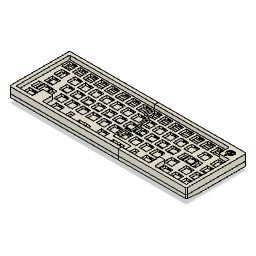
3d_print_case (Autodesk Fusion 360 design; units mm, degrees)
Autodesk Fusion 360 part; units mm, degrees
note: some values were not read from the file. Chosen so that the rebuilt part matches the saved one: which bodies a step acts on; which face or edge a step refers to. Set by a fixed rule: which sketch regions a step uses.
(part 1 of 3)
sketch "plate case top view" plane through (0, 0, 0) normal (0, 1, 0) x (1, 0, 0)
  line L0 (136.8258, 5.1029) -> (150.8248, 5.1029)
  line L1 (146.0628, 43.203) -> (132.0628, 43.203)
  line L2 (122.5378, 24.1528) -> (122.5378, 38.1522)
  line L3 (289.2258, 57.2023) -> (303.2248, 57.2023)
  line L4 (198.4498, 62.253) -> (184.4508, 62.253)
  line L5 (207.9748, 95.3023) -> (207.9748, 81.303)
  line L6 (284.1748, 95.3023) -> (284.1748, 81.303)
  line L7 (212.7378, 38.1522) -> (212.7378, 24.1528)
  line L8 (289.2258, 19.1023) -> (303.2248, 19.1023)
  line L9 (303.2248, 38.1522) -> (303.2248, 24.1528)
  line L10 (103.1998, 62.253) -> (89.2005, 62.253)
  line L11 (222.5508, 62.253) -> (222.5508, 76.2523)
  line L12 (231.7878, 19.1023) -> (231.7878, 5.1029)
  line L13 (265.1248, 95.3023) -> (265.1248, 81.303)
  line L14 (213.0258, 81.303) -> (213.0258, 95.3023)
  line L15 (303.2248, 62.253) -> (289.2258, 62.253)
  line L16 (193.9758, 81.303) -> (193.9758, 95.3023)
  line L17 (270.1758, 5.1029) -> (270.1758, 19.1023)
  line L18 (184.4508, 76.2523) -> (198.4498, 76.2523)
  line L19 (289.2258, 62.253) -> (289.2258, 76.2523)
  line L20 (246.0748, 95.3023) -> (246.0748, 81.303)
  line L21 (303.2248, 43.203) -> (289.2258, 43.203)
  line L22 (270.1758, 24.1528) -> (270.1758, 38.1522)
  line L23 (236.5498, 76.2523) -> (236.5498, 62.253)
  line L24 (79.6755, 95.3023) -> (93.6748, 95.3023)
  line L25 (179.3998, 76.2523) -> (179.3998, 62.253)
  line L26 (289.2258, 57.2023) -> (303.2248, 57.2023)
  line L27 (303.2248, 76.2523) -> (303.2248, 62.253)
  line L28 (203.2128, 43.203) -> (189.2128, 43.203)
  line L29 (188.9248, 95.3023) -> (188.9248, 81.303)
  line L30 (231.7878, 24.1528) -> (217.7878, 24.1528)
  line L31 (231.7878, 38.1522) -> (231.7878, 24.1528)
  line L32 (270.1758, 5.1029) -> (270.1758, 19.1023)
  line L33 (198.4498, 62.253) -> (184.4508, 62.253)
  line L34 (303.2248, 24.1528) -> (289.2258, 24.1528)
  line L35 (155.8758, 81.303) -> (155.8758, 95.3023)
  line L36 (217.7878, 38.1522) -> (231.7878, 38.1522)
  line L37 (203.5008, 76.2523) -> (217.4998, 76.2523)
  line L38 (232.0758, 81.303) -> (232.0758, 95.3023)
  line L39 (155.8758, 95.3023) -> (169.8748, 95.3023)
  line L40 (207.9748, 95.3023) -> (207.9748, 81.303)
  line L41 (284.1748, 5.1029) -> (270.1758, 5.1029)
  line L42 (284.1748, 19.1023) -> (284.1748, 5.1029)
  line L43 (189.2128, 57.2023) -> (203.2128, 57.2023)
  line L44 (303.2248, 62.253) -> (289.2258, 62.253)
  line L45 (303.2248, 5.1029) -> (289.2258, 5.1029)
  line L46 (241.6008, 76.2523) -> (255.5998, 76.2523)
  line L47 (222.5508, 62.253) -> (222.5508, 76.2523)
  line L48 (255.5998, 76.2523) -> (255.5998, 62.253)
  line L49 (289.2258, 62.253) -> (289.2258, 76.2523)
  line L50 (289.2258, 19.1023) -> (303.2248, 19.1023)
  line L51 (251.1258, 81.303) -> (251.1258, 95.3023)
  line L52 (270.1758, 81.303) -> (270.1758, 95.3023)
  line L53 (284.1748, 81.303) -> (270.1758, 81.303)
  line L54 (270.1758, 38.1522) -> (284.1748, 38.1522)
  line L55 (165.4008, 62.253) -> (165.4008, 76.2523)
  line L56 (303.2248, 5.1029) -> (289.2258, 5.1029)
  line L57 (251.1258, 81.303) -> (251.1258, 95.3023)
  line L58 (289.2258, 38.1522) -> (303.2248, 38.1522)
  line L59 (284.1748, 5.1029) -> (270.1758, 5.1029)
  line L60 (98.7241, 81.303) -> (98.7241, 95.3023)
  line L61 (270.1758, 19.1023) -> (284.1748, 19.1023)
  line L62 (89.2005, 76.2523) -> (103.1998, 76.2523)
  line L63 (79.6755, 81.303) -> (79.6755, 95.3023)
  line L64 (93.6748, 95.3023) -> (93.6748, 81.303)
  line L65 (93.6748, 81.303) -> (79.6755, 81.303)
  line L66 (255.5998, 62.253) -> (241.6008, 62.253)
  line L67 (270.1758, 95.3023) -> (284.1748, 95.3023)
  line L68 (188.9248, 81.303) -> (174.9258, 81.303)
  line L69 (289.2258, 24.1528) -> (289.2258, 38.1522)
  line L70 (265.4128, 62.253) -> (265.4128, 76.2523)
  line L71 (169.8748, 95.3023) -> (169.8748, 81.303)
  line L72 (74.913, 57.2023) -> (88.9123, 57.2023)
  line L73 (255.5998, 76.2523) -> (255.5998, 62.253)
  line L74 (207.9748, 81.303) -> (193.9758, 81.303)
  line L75 (270.1758, 19.1023) -> (284.1748, 19.1023)
  line L76 (289.2258, 5.1029) -> (289.2258, 19.1023)
  line L77 (279.4128, 62.253) -> (265.4128, 62.253)
  line L78 (222.2628, 43.203) -> (208.2628, 43.203)
  line L79 (265.4128, 62.253) -> (265.4128, 76.2523)
  line L80 (231.7878, 24.1528) -> (217.7878, 24.1528)
  line L81 (174.9258, 95.3023) -> (188.9248, 95.3023)
  line L82 (217.7878, 19.1023) -> (231.7878, 19.1023)
  line L83 (217.4998, 62.253) -> (203.5008, 62.253)
  line L84 (231.7878, 5.1029) -> (217.7878, 5.1029)
  line L85 (203.5008, 62.253) -> (203.5008, 76.2523)
  line L86 (155.8758, 95.3023) -> (169.8748, 95.3023)
  line L87 (217.4998, 62.253) -> (203.5008, 62.253)
  line L88 (231.7878, 5.1029) -> (217.7878, 5.1029)
  line L89 (303.2248, 76.2523) -> (303.2248, 62.253)
  line L90 (227.0248, 95.3023) -> (227.0248, 81.303)
  line L91 (284.1748, 19.1023) -> (284.1748, 5.1029)
  line L92 (279.4128, 76.2523) -> (279.4128, 62.253)
  line L93 (284.1748, 38.1522) -> (284.1748, 24.1528)
  line L94 (179.3998, 62.253) -> (165.4008, 62.253)
  line L95 (284.1748, 24.1528) -> (270.1758, 24.1528)
  line L96 (184.4508, 76.2523) -> (198.4498, 76.2523)
  line L97 (213.0258, 81.303) -> (213.0258, 95.3023)
  line L98 (198.4498, 76.2523) -> (198.4498, 62.253)
  line L99 (174.9258, 95.3023) -> (188.9248, 95.3023)
  line L100 (231.7878, 19.1023) -> (231.7878, 5.1029)
  line L101 (227.0248, 95.3023) -> (227.0248, 81.303)
  line L102 (289.2258, 76.2523) -> (303.2248, 76.2523)
  line L103 (208.2628, 57.2023) -> (222.2628, 57.2023)
  line L104 (174.9258, 81.303) -> (174.9258, 95.3023)
  line L105 (217.4998, 76.2523) -> (217.4998, 62.253)
  line L106 (212.7378, 24.1528) -> (198.7378, 24.1528)
  line L107 (93.6748, 95.3023) -> (93.6748, 81.303)
  line L108 (184.1628, 43.203) -> (170.1628, 43.203)
  line L109 (74.6248, 95.3023) -> (74.6248, 81.303)
  line L110 (103.1998, 62.253) -> (89.2005, 62.253)
  line L111 (79.6755, 81.303) -> (79.6755, 95.3023)
  line L112 (89.2005, 76.2523) -> (103.1998, 76.2523)
  line L113 (189.2128, 57.2023) -> (203.2128, 57.2023)
  line L114 (303.2248, 19.1023) -> (303.2248, 5.1029)
  line L115 (303.2248, 43.203) -> (289.2258, 43.203)
  line L116 (231.7878, 38.1522) -> (231.7878, 24.1528)
  line L117 (284.1748, 95.3023) -> (284.1748, 81.303)
  line L118 (217.4998, 76.2523) -> (217.4998, 62.253)
  line L119 (217.7878, 24.1528) -> (217.7878, 38.1522)
  line L120 (203.5008, 76.2523) -> (217.4998, 76.2523)
  line L121 (198.4498, 76.2523) -> (198.4498, 62.253)
  line L122 (279.4128, 62.253) -> (265.4128, 62.253)
  line L123 (213.0258, 95.3023) -> (227.0248, 95.3023)
  line L124 (217.7878, 19.1023) -> (231.7878, 19.1023)
  line L125 (289.2258, 76.2523) -> (303.2248, 76.2523)
  line L126 (169.8748, 95.3023) -> (169.8748, 81.303)
  line L127 (227.0248, 81.303) -> (213.0258, 81.303)
  line L128 (265.4128, 76.2523) -> (279.4128, 76.2523)
  line L129 (203.5008, 62.253) -> (203.5008, 76.2523)
  line L130 (169.8748, 81.303) -> (155.8758, 81.303)
  line L131 (169.8748, 81.303) -> (155.8758, 81.303)
  line L132 (212.7378, 38.1522) -> (212.7378, 24.1528)
  line L133 (265.1248, 95.3023) -> (265.1248, 81.303)
  line L134 (174.9258, 81.303) -> (174.9258, 95.3023)
  line L135 (303.2248, 38.1522) -> (303.2248, 24.1528)
  line L136 (212.7378, 24.1528) -> (198.7378, 24.1528)
  line L137 (246.0748, 95.3023) -> (246.0748, 81.303)
  line L138 (179.3998, 76.2523) -> (179.3998, 62.253)
  line L139 (303.2248, 19.1023) -> (303.2248, 5.1029)
  line L140 (193.9758, 95.3023) -> (207.9748, 95.3023)
  line L141 (289.2258, 5.1029) -> (289.2258, 19.1023)
  line L142 (155.8758, 81.303) -> (155.8758, 95.3023)
  line L143 (217.7878, 24.1528) -> (217.7878, 38.1522)
  line L144 (213.0258, 95.3023) -> (227.0248, 95.3023)
  line L145 (188.9248, 81.303) -> (174.9258, 81.303)
  line L146 (188.9248, 95.3023) -> (188.9248, 81.303)
  line L147 (270.1758, 81.303) -> (270.1758, 95.3023)
  line L148 (89.2005, 62.253) -> (89.2005, 76.2523)
  line L149 (74.913, 57.2023) -> (88.9123, 57.2023)
  line L150 (284.1748, 38.1522) -> (284.1748, 24.1528)
  line L151 (241.6008, 76.2523) -> (255.5998, 76.2523)
  line L152 (303.2248, 24.1528) -> (289.2258, 24.1528)
  line L153 (265.4128, 76.2523) -> (279.4128, 76.2523)
  line L154 (284.1748, 81.303) -> (270.1758, 81.303)
  line L155 (222.2628, 43.203) -> (208.2628, 43.203)
  line L156 (217.7878, 5.1029) -> (217.7878, 19.1023)
  line L157 (227.0248, 81.303) -> (213.0258, 81.303)
  line L158 (208.2628, 57.2023) -> (222.2628, 57.2023)
  line L159 (193.9758, 81.303) -> (193.9758, 95.3023)
  line L160 (279.4128, 76.2523) -> (279.4128, 62.253)
  line L161 (217.7878, 38.1522) -> (231.7878, 38.1522)
  line L162 (232.0758, 81.303) -> (232.0758, 95.3023)
  line L163 (217.7878, 5.1029) -> (217.7878, 19.1023)
  line L164 (270.1758, 95.3023) -> (284.1748, 95.3023)
  line L165 (255.5998, 62.253) -> (241.6008, 62.253)
  line L166 (198.7378, 38.1522) -> (212.7378, 38.1522)
  line L167 (170.1628, 57.2023) -> (184.1628, 57.2023)
  line L168 (203.2128, 43.203) -> (189.2128, 43.203)
  line L169 (89.2005, 62.253) -> (89.2005, 76.2523)
  line L170 (131.7748, 81.303) -> (117.7738, 81.303)
  line L171 (127.3008, 76.2523) -> (141.2998, 76.2523)
  line L172 (132.0628, 57.2023) -> (146.0628, 57.2023)
  line L173 (50.8123, 57.2023) -> (50.8123, 43.203)
  line L174 (108.2508, 62.253) -> (108.2508, 76.2523)
  line L175 (10.6178, 43.203) -> (10.6178, 57.2023)
  line L176 (69.8623, 5.1029) -> (55.863, 5.1029)
  line L177 (170.1628, 43.203) -> (170.1628, 57.2023)
  line L178 (107.9628, 57.2023) -> (107.9628, 43.203)
  line L179 (22.5255, 95.3023) -> (36.5248, 95.3023)
  line L180 (107.9628, 43.203) -> (93.963, 43.203)
  line L181 (46.338, 24.1528) -> (46.338, 38.1522)
  line L182 (88.9123, 57.2023) -> (88.9123, 43.203)
  line L183 (184.1628, 57.2023) -> (184.1628, 43.203)
  line L184 (51.1005, 62.253) -> (51.1005, 76.2523)
  line L185 (112.7248, 81.303) -> (98.7241, 81.303)
  line L186 (112.7248, 81.303) -> (98.7241, 81.303)
  line L187 (193.6878, 38.1522) -> (193.6878, 24.1528)
  line L188 (3.4754, 95.3023) -> (17.475, 95.3023)
  line L189 (289.2258, 24.1528) -> (289.2258, 38.1522)
  line L190 (241.6008, 62.253) -> (241.6008, 76.2523)
  line L191 (160.6378, 38.1522) -> (174.6378, 38.1522)
  line L192 (22.2375, 76.2523) -> (22.2375, 62.253)
  line L193 (243.9818, 24.1528) -> (243.9818, 38.1522)
  line L194 (65.0998, 76.2523) -> (65.0998, 62.253)
  line L195 (50.8123, 57.2023) -> (50.8123, 43.203)
  line L196 (32.0505, 62.253) -> (32.0505, 76.2523)
  line L197 (22.2375, 76.2523) -> (22.2375, 62.253)
  line L198 (65.0998, 76.2523) -> (65.0998, 62.253)
  line L199 (251.1258, 19.1023) -> (265.1248, 19.1023)
  line L200 (55.863, 57.2023) -> (69.8623, 57.2023)
  line L201 (22.5255, 81.303) -> (22.5255, 95.3023)
  line L202 (122.2498, 76.2523) -> (122.2498, 62.253)
  line L203 (243.9818, 38.1522) -> (257.9808, 38.1522)
  line L204 (55.5748, 81.303) -> (41.5755, 81.303)
  line L205 (29.3812, 38.1522) -> (15.3817, 38.1522)
  line L206 (60.3373, 24.1528) -> (46.338, 24.1528)
  line L207 (303.2248, 57.2023) -> (303.2248, 43.203)
  line L208 (165.1128, 57.2023) -> (165.1128, 43.203)
  line L209 (69.8623, 19.1023) -> (69.8623, 5.1029)
  line L210 (222.2628, 57.2023) -> (222.2628, 43.203)
  line L211 (55.863, 5.1029) -> (55.863, 19.1023)
  line L212 (46.338, 38.1522) -> (60.3373, 38.1522)
  line L213 (36.813, 57.2023) -> (50.8123, 57.2023)
  line L214 (170.1628, 43.203) -> (170.1628, 57.2023)
  line L215 (117.7738, 81.303) -> (117.7738, 95.3023)
  line L216 (303.2248, 57.2023) -> (303.2248, 43.203)
  line L217 (127.0128, 43.203) -> (113.0128, 43.203)
  line L218 (60.6255, 81.303) -> (60.6255, 95.3023)
  line L219 (265.1248, 19.1023) -> (265.1248, 5.1029)
  line L220 (132.0628, 57.2023) -> (146.0628, 57.2023)
  line L221 (32.0505, 76.2523) -> (46.0498, 76.2523)
  line L222 (222.2628, 57.2023) -> (222.2628, 43.203)
  line L223 (8.2379, 19.1023) -> (22.2375, 19.1023)
  line L224 (98.7241, 95.3023) -> (112.7248, 95.3023)
  line L225 (146.3508, 62.253) -> (146.3508, 76.2523)
  line L226 (222.5508, 76.2523) -> (236.5498, 76.2523)
  line L227 (65.388, 38.1522) -> (79.3873, 38.1522)
  line L228 (236.5498, 62.253) -> (222.5508, 62.253)
  line L229 (232.0758, 95.3023) -> (246.0748, 95.3023)
  line L230 (74.6248, 81.303) -> (60.6255, 81.303)
  line L231 (17.475, 95.3023) -> (17.475, 81.303)
  line L232 (265.1248, 5.1029) -> (251.1258, 5.1029)
  line L233 (184.1628, 57.2023) -> (184.1628, 43.203)
  line L234 (55.863, 5.1029) -> (55.863, 19.1023)
  line L235 (127.3008, 62.253) -> (127.3008, 76.2523)
  line L236 (113.0128, 57.2023) -> (127.0128, 57.2023)
  line L237 (36.813, 43.203) -> (36.813, 57.2023)
  line L238 (22.2375, 19.1023) -> (22.2375, 5.1029)
  line L239 (122.2498, 62.253) -> (108.2508, 62.253)
  line L240 (141.2998, 62.253) -> (127.3008, 62.253)
  line L241 (193.6878, 38.1522) -> (193.6878, 24.1528)
  line L242 (122.2498, 62.253) -> (108.2508, 62.253)
  line L243 (103.4878, 38.1522) -> (117.4878, 38.1522)
  line L244 (207.9748, 81.303) -> (193.9758, 81.303)
  line L245 (198.7378, 38.1522) -> (212.7378, 38.1522)
  line L246 (150.8248, 95.3023) -> (150.8248, 81.303)
  line L247 (146.3508, 76.2523) -> (160.3498, 76.2523)
  line L248 (127.0128, 43.203) -> (113.0128, 43.203)
  line L249 (236.5498, 62.253) -> (222.5508, 62.253)
  line L250 (79.3873, 24.1528) -> (65.388, 24.1528)
  line L251 (74.913, 43.203) -> (74.913, 57.2023)
  line L252 (246.0748, 81.303) -> (232.0758, 81.303)
  line L253 (74.913, 43.203) -> (74.913, 57.2023)
  line L254 (0.9508, 2.5769) -> (0.9508, 97.8267)
  line L255 (241.3128, 43.203) -> (227.3128, 43.203)
  line L256 (146.0628, 57.2023) -> (146.0628, 43.203)
  line L257 (151.1128, 43.203) -> (151.1128, 57.2023)
  line L258 (107.9628, 57.2023) -> (107.9628, 43.203)
  line L259 (246.0748, 81.303) -> (232.0758, 81.303)
  line L260 (227.3128, 57.2023) -> (241.3128, 57.2023)
  line L261 (232.0758, 95.3023) -> (246.0748, 95.3023)
  line L262 (127.0128, 57.2023) -> (127.0128, 43.203)
  line L263 (0.9508, 2.5769) -> (0.9508, 97.8267)
  line L264 (151.1128, 43.203) -> (151.1128, 57.2023)
  line L265 (227.3128, 43.203) -> (227.3128, 57.2023)
  line L266 (46.0498, 62.253) -> (32.0505, 62.253)
  line L267 (113.0128, 43.203) -> (113.0128, 57.2023)
  line L268 (93.963, 43.203) -> (93.963, 57.2023)
  line L269 (203.2128, 57.2023) -> (203.2128, 43.203)
  line L270 (36.5248, 81.303) -> (22.5255, 81.303)
  line L271 (257.9808, 38.1522) -> (257.9808, 24.1528)
  line L272 (165.4008, 76.2523) -> (179.3998, 76.2523)
  line L273 (65.388, 24.1528) -> (65.388, 38.1522)
  line L274 (103.4878, 38.1522) -> (117.4878, 38.1522)
  line L275 (79.6755, 95.3023) -> (93.6748, 95.3023)
  line L276 (165.4008, 76.2523) -> (179.3998, 76.2523)
  line L277 (93.963, 57.2023) -> (107.9628, 57.2023)
  line L278 (136.8258, 95.3023) -> (150.8248, 95.3023)
  line L279 (84.1498, 76.2523) -> (84.1498, 62.253)
  line L280 (127.3008, 76.2523) -> (141.2998, 76.2523)
  line L281 (160.3498, 76.2523) -> (160.3498, 62.253)
  line L282 (8.2379, 62.253) -> (8.2379, 76.2523)
  line L283 (22.2375, 62.253) -> (8.2379, 62.253)
  line L284 (155.5878, 38.1522) -> (155.5878, 24.1528)
  line L285 (55.863, 19.1023) -> (69.8623, 19.1023)
  line L286 (55.863, 57.2023) -> (69.8623, 57.2023)
  line L287 (8.2379, 76.2523) -> (22.2375, 76.2523)
  line L288 (24.6187, 57.2023) -> (24.6187, 43.203)
  line L289 (60.3373, 38.1522) -> (60.3373, 24.1528)
  line L290 (208.2628, 43.203) -> (208.2628, 57.2023)
  line L291 (127.3008, 62.253) -> (127.3008, 76.2523)
  line L292 (46.0498, 76.2523) -> (46.0498, 62.253)
  line L293 (136.5378, 24.1528) -> (122.5378, 24.1528)
  line L294 (265.1248, 81.303) -> (251.1258, 81.303)
  line L295 (22.5255, 81.303) -> (22.5255, 95.3023)
  line L296 (208.2628, 43.203) -> (208.2628, 57.2023)
  line L297 (55.5748, 81.303) -> (41.5755, 81.303)
  line L298 (60.6255, 95.3023) -> (74.6248, 95.3023)
  line L299 (241.3128, 43.203) -> (227.3128, 43.203)
  line L300 (41.5755, 95.3023) -> (55.5748, 95.3023)
  line L301 (193.6878, 24.1528) -> (179.6878, 24.1528)
  line L302 (24.6187, 43.203) -> (10.6178, 43.203)
  line L303 (65.0998, 62.253) -> (51.1005, 62.253)
  line L304 (222.5508, 76.2523) -> (236.5498, 76.2523)
  line L305 (65.388, 38.1522) -> (79.3873, 38.1522)
  line L306 (189.2128, 43.203) -> (189.2128, 57.2023)
  line L307 (69.8623, 19.1023) -> (69.8623, 5.1029)
  line L308 (193.9758, 95.3023) -> (207.9748, 95.3023)
  line L309 (136.8258, 81.303) -> (136.8258, 95.3023)
  line L310 (227.3128, 43.203) -> (227.3128, 57.2023)
  line L311 (117.7738, 95.3023) -> (131.7748, 95.3023)
  line L312 (108.2508, 76.2523) -> (122.2498, 76.2523)
  line L313 (65.0998, 62.253) -> (51.1005, 62.253)
  line L314 (198.7378, 24.1528) -> (198.7378, 38.1522)
  line L315 (243.9818, 38.1522) -> (257.9808, 38.1522)
  line L316 (69.8623, 57.2023) -> (69.8623, 43.203)
  line L317 (8.2379, 19.1023) -> (22.2375, 19.1023)
  line L318 (179.6878, 38.1522) -> (193.6878, 38.1522)
  line L319 (165.4008, 62.253) -> (165.4008, 76.2523)
  line L320 (103.1998, 76.2523) -> (103.1998, 62.253)
  line L321 (55.863, 43.203) -> (55.863, 57.2023)
  line L322 (22.2375, 5.1029) -> (8.2379, 5.1029)
  line L323 (122.5378, 24.1528) -> (122.5378, 38.1522)
  line L324 (160.3498, 62.253) -> (146.3508, 62.253)
  line L325 (146.3508, 76.2523) -> (160.3498, 76.2523)
  line L326 (0.9508, 97.8267) -> (305.7508, 97.8267)
  line L327 (305.7508, 2.5769) -> (0.9508, 2.5769)
  line L328 (165.1128, 43.203) -> (151.1128, 43.203)
  line L329 (305.7508, 2.5769) -> (0.9508, 2.5769)
  line L330 (155.5878, 24.1528) -> (141.5878, 24.1528)
  line L331 (70.1505, 76.2523) -> (84.1498, 76.2523)
  line L332 (151.1128, 57.2023) -> (165.1128, 57.2023)
  line L333 (141.5878, 38.1522) -> (155.5878, 38.1522)
  line L334 (50.8123, 43.203) -> (36.813, 43.203)
  line L335 (136.5378, 24.1528) -> (122.5378, 24.1528)
  line L336 (179.6878, 24.1528) -> (179.6878, 38.1522)
  line L337 (36.5248, 81.303) -> (22.5255, 81.303)
  line L338 (127.0128, 57.2023) -> (127.0128, 43.203)
  line L339 (131.7748, 95.3023) -> (131.7748, 81.303)
  line L340 (136.8258, 81.303) -> (136.8258, 95.3023)
  line L341 (60.6255, 81.303) -> (60.6255, 95.3023)
  line L342 (251.1258, 5.1029) -> (251.1258, 19.1023)
  line L343 (8.2379, 5.1029) -> (8.2379, 19.1023)
  line L344 (60.3373, 24.1528) -> (46.338, 24.1528)
  line L345 (46.338, 38.1522) -> (60.3373, 38.1522)
  line L346 (198.7378, 24.1528) -> (198.7378, 38.1522)
  line L347 (257.9808, 38.1522) -> (257.9808, 24.1528)
  line L348 (117.7738, 95.3023) -> (131.7748, 95.3023)
  line L349 (241.3128, 57.2023) -> (241.3128, 43.203)
  line L350 (132.0628, 43.203) -> (132.0628, 57.2023)
  line L351 (98.7241, 81.303) -> (98.7241, 95.3023)
  line L352 (179.3998, 62.253) -> (165.4008, 62.253)
  line L353 (15.3817, 24.1528) -> (29.3812, 24.1528)
  line L354 (251.1258, 95.3023) -> (265.1248, 95.3023)
  line L355 (70.1505, 62.253) -> (70.1505, 76.2523)
  line L356 (151.1128, 57.2023) -> (165.1128, 57.2023)
  line L357 (55.863, 19.1023) -> (69.8623, 19.1023)
  line L358 (41.5755, 81.303) -> (41.5755, 95.3023)
  line L359 (258.2678, 43.203) -> (272.2688, 43.203)
  line L360 (41.5755, 95.3023) -> (55.5748, 95.3023)
  line L361 (150.8248, 81.303) -> (136.8258, 81.303)
  line L362 (117.4878, 38.1522) -> (117.4878, 24.1528)
  line L363 (22.2375, 19.1023) -> (22.2375, 5.1029)
  line L364 (284.1748, 24.1528) -> (270.1758, 24.1528)
  line L365 (103.1998, 76.2523) -> (103.1998, 62.253)
  line L366 (93.963, 43.203) -> (93.963, 57.2023)
  line L367 (251.1258, 19.1023) -> (265.1248, 19.1023)
  line L368 (113.0128, 57.2023) -> (127.0128, 57.2023)
  line L369 (8.2379, 62.253) -> (8.2379, 76.2523)
  line L370 (69.8623, 57.2023) -> (69.8623, 43.203)
  line L371 (117.4878, 24.1528) -> (103.4878, 24.1528)
  line L372 (272.2688, 57.2023) -> (258.2678, 57.2023)
  line L373 (265.1248, 19.1023) -> (265.1248, 5.1029)
  line L374 (122.2498, 76.2523) -> (122.2498, 62.253)
  line L375 (193.6878, 24.1528) -> (179.6878, 24.1528)
  line L376 (257.9808, 24.1528) -> (243.9818, 24.1528)
  line L377 (17.475, 81.303) -> (3.4754, 81.303)
  line L378 (108.2508, 76.2523) -> (122.2498, 76.2523)
  line L379 (36.5248, 95.3023) -> (36.5248, 81.303)
  line L380 (146.3508, 62.253) -> (146.3508, 76.2523)
  line L381 (60.3373, 38.1522) -> (60.3373, 24.1528)
  line L382 (46.0498, 62.253) -> (32.0505, 62.253)
  line L383 (203.2128, 57.2023) -> (203.2128, 43.203)
  line L384 (179.6878, 38.1522) -> (193.6878, 38.1522)
  line L385 (174.6378, 24.1528) -> (160.6378, 24.1528)
  line L386 (107.9628, 43.203) -> (93.963, 43.203)
  line L387 (10.6178, 57.2023) -> (24.6187, 57.2023)
  line L388 (174.6378, 38.1522) -> (174.6378, 24.1528)
  line L389 (55.5748, 95.3023) -> (55.5748, 81.303)
  line L390 (36.813, 57.2023) -> (50.8123, 57.2023)
  line L391 (305.7508, 97.8267) -> (305.7508, 2.5769)
  line L392 (251.1258, 5.1029) -> (251.1258, 19.1023)
  line L393 (22.2375, 5.1029) -> (8.2379, 5.1029)
  line L394 (113.0128, 43.203) -> (113.0128, 57.2023)
  line L395 (88.9123, 57.2023) -> (88.9123, 43.203)
  line L396 (70.1505, 62.253) -> (70.1505, 76.2523)
  line L397 (305.7508, 97.8267) -> (305.7508, 2.5769)
  line L398 (32.0505, 76.2523) -> (46.0498, 76.2523)
  line L399 (98.7241, 95.3023) -> (112.7248, 95.3023)
  line L400 (174.6378, 24.1528) -> (160.6378, 24.1528)
  line L401 (15.3817, 24.1528) -> (29.3812, 24.1528)
  line L402 (69.8623, 43.203) -> (55.863, 43.203)
  line L403 (160.6378, 24.1528) -> (160.6378, 38.1522)
  line L404 (189.2128, 43.203) -> (189.2128, 57.2023)
  line L405 (174.6378, 38.1522) -> (174.6378, 24.1528)
  line L406 (79.3873, 24.1528) -> (65.388, 24.1528)
  line L407 (51.1005, 62.253) -> (51.1005, 76.2523)
  line L408 (55.863, 43.203) -> (55.863, 57.2023)
  line L409 (84.1498, 62.253) -> (70.1505, 62.253)
  line L410 (84.1498, 62.253) -> (70.1505, 62.253)
  line L411 (141.2998, 76.2523) -> (141.2998, 62.253)
  line L412 (17.475, 95.3023) -> (17.475, 81.303)
  line L413 (289.2258, 43.203) -> (289.2258, 57.2023)
  line L414 (258.2678, 43.203) -> (272.2688, 43.203)
  line L415 (60.6255, 95.3023) -> (74.6248, 95.3023)
  line L416 (70.1505, 76.2523) -> (84.1498, 76.2523)
  line L417 (46.338, 24.1528) -> (46.338, 38.1522)
  line L418 (146.0628, 57.2023) -> (146.0628, 43.203)
  line L419 (22.5255, 95.3023) -> (36.5248, 95.3023)
  line L420 (69.8623, 5.1029) -> (55.863, 5.1029)
  line L421 (3.4754, 81.303) -> (3.4754, 95.3023)
  line L422 (17.475, 81.303) -> (3.4754, 81.303)
  line L423 (8.2379, 76.2523) -> (22.2375, 76.2523)
  line L424 (289.2258, 43.203) -> (289.2258, 57.2023)
  line L425 (29.3812, 38.1522) -> (15.3817, 38.1522)
  line L426 (141.2998, 76.2523) -> (141.2998, 62.253)
  line L427 (131.7748, 81.303) -> (117.7738, 81.303)
  line L428 (46.0498, 76.2523) -> (46.0498, 62.253)
  line L429 (10.6178, 43.203) -> (10.6178, 57.2023)
  line L430 (160.6378, 38.1522) -> (174.6378, 38.1522)
  line L431 (65.388, 24.1528) -> (65.388, 38.1522)
  line L432 (8.2379, 5.1029) -> (8.2379, 19.1023)
  line L433 (272.2688, 57.2023) -> (258.2678, 57.2023)
  line L434 (112.7248, 95.3023) -> (112.7248, 81.303)
  line L435 (108.2508, 62.253) -> (108.2508, 76.2523)
  line L436 (112.7248, 95.3023) -> (112.7248, 81.303)
  line L437 (117.7738, 81.303) -> (117.7738, 95.3023)
  line L438 (289.2258, 38.1522) -> (303.2248, 38.1522)
  line L439 (55.5748, 95.3023) -> (55.5748, 81.303)
  line L440 (3.4754, 95.3023) -> (17.475, 95.3023)
  line L441 (24.6187, 43.203) -> (10.6178, 43.203)
  line L442 (69.8623, 43.203) -> (55.863, 43.203)
  line L443 (251.1258, 95.3023) -> (265.1248, 95.3023)
  line L444 (160.3498, 76.2523) -> (160.3498, 62.253)
  line L445 (170.1628, 57.2023) -> (184.1628, 57.2023)
  line L446 (141.2998, 62.253) -> (127.3008, 62.253)
  line L447 (74.6248, 81.303) -> (60.6255, 81.303)
  line L448 (227.3128, 57.2023) -> (241.3128, 57.2023)
  line L449 (122.5378, 38.1522) -> (136.5378, 38.1522)
  line L450 (3.4754, 81.303) -> (3.4754, 95.3023)
  line L451 (36.5248, 95.3023) -> (36.5248, 81.303)
  line L452 (36.813, 43.203) -> (36.813, 57.2023)
  line L453 (22.2375, 62.253) -> (8.2379, 62.253)
  line L454 (243.9818, 24.1528) -> (243.9818, 38.1522)
  line L455 (165.1128, 57.2023) -> (165.1128, 43.203)
  line L456 (51.1005, 76.2523) -> (65.0998, 76.2523)
  line L457 (150.8248, 95.3023) -> (150.8248, 81.303)
  line L458 (155.5878, 38.1522) -> (155.5878, 24.1528)
  line L459 (165.1128, 43.203) -> (151.1128, 43.203)
  line L460 (160.6378, 24.1528) -> (160.6378, 38.1522)
  line L461 (10.6178, 57.2023) -> (24.6187, 57.2023)
  line L462 (117.4878, 24.1528) -> (103.4878, 24.1528)
  line L463 (50.8123, 43.203) -> (36.813, 43.203)
  line L464 (184.4508, 62.253) -> (184.4508, 76.2523)
  line L465 (179.6878, 24.1528) -> (179.6878, 38.1522)
  line L466 (93.6748, 81.303) -> (79.6755, 81.303)
  line L467 (32.0505, 62.253) -> (32.0505, 76.2523)
  line L468 (117.4878, 38.1522) -> (117.4878, 24.1528)
  line L469 (131.7748, 95.3023) -> (131.7748, 81.303)
  line L470 (150.8248, 81.303) -> (136.8258, 81.303)
  line L471 (241.6008, 62.253) -> (241.6008, 76.2523)
  line L472 (74.6248, 95.3023) -> (74.6248, 81.303)
  line L473 (84.1498, 76.2523) -> (84.1498, 62.253)
  line L474 (132.0628, 43.203) -> (132.0628, 57.2023)
  line L475 (241.3128, 57.2023) -> (241.3128, 43.203)
  line L476 (257.9808, 24.1528) -> (243.9818, 24.1528)
  line L477 (24.6187, 57.2023) -> (24.6187, 43.203)
  line L478 (270.1758, 24.1528) -> (270.1758, 38.1522)
  line L479 (236.5498, 76.2523) -> (236.5498, 62.253)
  line L480 (184.1628, 43.203) -> (170.1628, 43.203)
  line L481 (41.5755, 81.303) -> (41.5755, 95.3023)
  line L482 (265.1248, 81.303) -> (251.1258, 81.303)
  line L483 (136.8258, 95.3023) -> (150.8248, 95.3023)
  line L484 (93.963, 57.2023) -> (107.9628, 57.2023)
  line L485 (51.1005, 76.2523) -> (65.0998, 76.2523)
  line L486 (270.1758, 38.1522) -> (284.1748, 38.1522)
  line L487 (184.4508, 62.253) -> (184.4508, 76.2523)
  line L488 (265.1248, 5.1029) -> (251.1258, 5.1029)
  line L489 (155.5878, 24.1528) -> (141.5878, 24.1528)
  line L490 (136.5378, 38.1522) -> (136.5378, 24.1528)
  line L491 (136.8258, 5.1029) -> (150.8248, 5.1029)
  line L492 (150.8248, 19.1023) -> (136.8258, 19.1023)
  line L493 (84.438, 38.1522) -> (98.4373, 38.1522)
  line L494 (146.0628, 43.203) -> (132.0628, 43.203)
  line L495 (98.4373, 38.1522) -> (98.4373, 24.1528)
  line L496 (88.9123, 43.203) -> (74.913, 43.203)
  line L497 (141.5878, 24.1528) -> (141.5878, 38.1522)
  line L498 (79.3873, 38.1522) -> (79.3873, 24.1528)
  line L499 (150.8248, 19.1023) -> (136.8258, 19.1023)
  line L500 (136.5378, 38.1522) -> (136.5378, 24.1528)
  line L501 (122.5378, 38.1522) -> (136.5378, 38.1522)
  line L502 (84.438, 24.1528) -> (84.438, 38.1522)
  line L503 (98.4373, 24.1528) -> (84.438, 24.1528)
  line L504 (98.4373, 38.1522) -> (98.4373, 24.1528)
  line L505 (84.438, 24.1528) -> (84.438, 38.1522)
  line L506 (141.5878, 24.1528) -> (141.5878, 38.1522)
  line L507 (84.438, 38.1522) -> (98.4373, 38.1522)
  line L508 (103.4878, 24.1528) -> (103.4878, 38.1522)
  line L509 (79.3873, 38.1522) -> (79.3873, 24.1528)
  line L510 (0.9508, 97.8267) -> (305.7508, 97.8267)
  line L511 (103.4878, 24.1528) -> (103.4878, 38.1522)
  line L512 (88.9123, 43.203) -> (74.913, 43.203)
  line L513 (160.3498, 62.253) -> (146.3508, 62.253)
  line L514 (141.5878, 38.1522) -> (155.5878, 38.1522)
  line L515 (98.4373, 24.1528) -> (84.438, 24.1528)
  line L516 (13.8562, 37.604) -> (13.8562, 23.4018)
  line L517 (6.2811, 23.4018) -> (6.2811, 37.604)
  line L518 (15.3817, 38.1522) -> (15.3817, 24.1528)
  line L519 (6.2811, 37.604) -> (13.8562, 37.604)
  line L520 (6.2811, 23.4018) -> (13.8562, 23.4018)
  line L521 (30.9067, 37.604) -> (38.4817, 37.604)
  line L522 (38.4817, 37.604) -> (38.4817, 23.4018)
  line L523 (30.9067, 23.4018) -> (30.9067, 37.604)
  line L524 (29.3812, 38.1522) -> (29.3812, 24.1528)
  line L525 (30.9067, 23.4018) -> (38.4817, 23.4018)
  line L526 (256.7438, 56.6526) -> (256.7438, 42.4519)
  line L527 (256.7438, 42.4519) -> (249.1688, 42.4519)
  line L528 (249.1688, 42.4519) -> (249.1688, 56.6526)
  line L529 (258.2678, 57.2023) -> (258.2678, 43.203)
  line L530 (249.1688, 56.6526) -> (256.7438, 56.6526)
  line L531 (281.3678, 56.6526) -> (273.7928, 56.6526)
  line L532 (273.7928, 56.6526) -> (273.7928, 42.4519)
  line L533 (273.7928, 42.4519) -> (281.3678, 42.4519)
  line L534 (281.3678, 42.4519) -> (281.3678, 56.6526)
  line L535 (272.2688, 57.2023) -> (272.2688, 43.203)
  line L536 (205.1748, 18.5539) -> (197.5998, 18.5539)
  line L537 (197.5998, 18.5539) -> (197.5998, 4.3518)
  line L538 (197.5998, 4.3518) -> (205.1748, 4.3518)
  line L539 (205.1748, 4.3518) -> (205.1748, 18.5539)
  line L540 (82.4755, 18.5539) -> (90.0507, 18.5539)
  line L541 (90.0507, 18.5539) -> (90.0507, 4.3518)
  line L542 (90.0507, 4.3518) -> (82.4755, 4.3518)
  line L543 (82.4755, 4.3518) -> (82.4755, 18.5539)
  line L544 (150.8248, 19.1023) -> (150.8248, 5.1029)
  line L545 (136.8258, 19.1023) -> (136.8258, 5.1029)
  circle A0 centre (113.4382, 11.4529) radius 3
  line L546 (123.4382, 11.4529) -> (123.4382, 13.4529)
  line L547 (123.4382, 13.4529) -> (113.4382, 13.4529)
  line L548 (123.4382, 11.4529) -> (123.4382, 9.4529)
  line L549 (123.4382, 9.4529) -> (113.4382, 9.4529)
  line L550 (103.4382, 11.4529) -> (103.4382, 13.4529)
  line L551 (103.4382, 13.4529) -> (113.4382, 13.4529)
  line L552 (103.4382, 11.4529) -> (103.4382, 9.4529)
  line L553 (103.4382, 9.4529) -> (113.4382, 9.4529)
  line L554 (184.2123, 13.4529) -> (174.2123, 13.4529)
  line L555 (164.2123, 13.4529) -> (174.2123, 13.4529)
  line L556 (164.2123, 11.4529) -> (164.2123, 9.4529)
  line L557 (164.2123, 11.4529) -> (164.2123, 13.4529)
  line L558 (164.2123, 9.4529) -> (174.2123, 9.4529)
  line L559 (184.2123, 11.4529) -> (184.2123, 9.4529)
  circle A1 centre (174.2123, 11.4529) radius 3
  line L560 (184.2123, 9.4529) -> (174.2123, 9.4529)
  line L561 (184.2123, 11.4529) -> (184.2123, 13.4529)
  line L562 (306.1758, 2.1519) -> (0.5258, 2.1519)
  line L563 (0.5258, 2.1519) -> (0.5258, 98.2517)
  line L564 (0.5258, 98.2517) -> (306.1758, 98.2517)
  line L565 (306.1758, 98.2517) -> (306.1758, 2.1519)
  line L566 (312.1758, -3.8481) -> (-5.4742, -3.8481)
  line L567 (-5.4742, -3.8481) -> (-5.4742, 104.2517)
  line L568 (-5.4742, 104.2517) -> (312.1758, 104.2517)
  line L569 (312.1758, 104.2517) -> (312.1758, -3.8481)
  line L570 (30.0505, 3.1029) -> (30.0505, 21.1023)
  line L571 (30.0505, 21.1023) -> (48.0498, 21.1023)
  line L572 (48.0498, 21.1023) -> (48.0498, 3.1029)
  line L573 (30.0505, 3.1029) -> (30.0505, 2.1519)
  line L574 (48.0498, 3.1029) -> (48.0498, 2.1519)
  line L575 (249.1258, 21.1023) -> (239.6008, 21.1023)
  line L576 (239.6008, 21.1023) -> (239.6008, 2.1519)
  line L577 (249.1258, 21.1023) -> (249.1258, 2.1519)
  line L578 (287.2258, 98.2517) -> (306.1758, 98.2517)
  line L579 (306.1758, 98.2517) -> (306.1758, 79.303)
  line L580 (306.1758, 79.303) -> (287.2258, 79.303)
  line L581 (287.2258, 79.303) -> (287.2258, 98.2517)
  constraint coincident L562 L573.end
  constraint coincident L562 L574.end
  constraint coincident L562 L576.end
  constraint coincident L562 L577.end
  constraint coincident L565 L579.end
  constraint coincident L564 L578.start
extrude "Extrude1" add sketch "plate case top view" against normal blind 4 contours L254 L263 L326 L327 L329 L510 L562 L563 L564 L573 L581 | L254 L263 L326 L327 L329 L391 L397 L510 L570 L571 L572 L573 L574 L575 L576 L577 L580 L581 | L327 L329 L570 L571 L572 L573 L574 | L327 L329 L562 L573 L574 | L326 L391 L397 L510 L564 L565 L578 L579 L580 L581 | L326 L391 L397 L510 L580 L581 | L327 L329 L562 L574 L576 | L327 L329 L575 L576 L577 | L327 L329 L562 L576 L577 | L327 L329 L391 L397 L562 L565 L577 L580 | L566 L567 L568 L569 makes body 1
extrude "Extrude2" add sketch "plate case top view" along normal blind 7 contours L327 L329 L570 L571 L572 L573 L574 | L327 L329 L562 L573 L574 | L326 L391 L397 L510 L564 L565 L578 L579 L580 L581 | L326 L391 L397 L510 L580 L581 | L327 L329 L575 L576 L577 | L327 L329 L562 L576 L577 | L566 L567 L568 L569 bodies 1
sketch "plate switch clips" plane through (0, -4, 0) normal (0, -1, 0) x (1, 0, 0)
  line L0 (98.4373, -24.1528) -> (98.4373, -38.1522)
  line L1 (98.4373, -38.1522) -> (84.438, -38.1522)
  line L2 (84.438, -38.1522) -> (84.438, -24.1528)
  line L3 (84.438, -24.1528) -> (98.4373, -24.1528)
  line L4 (3.4754, -81.303) -> (17.475, -81.303)
  line L5 (17.475, -81.303) -> (17.475, -95.3023)
  line L6 (17.475, -95.3023) -> (3.4754, -95.3023)
  line L7 (3.4754, -95.3023) -> (3.4754, -81.303)
  line L8 (279.4128, -76.2523) -> (265.4128, -76.2523)
  line L9 (265.4128, -76.2523) -> (265.4128, -62.253)
  line L10 (265.4128, -62.253) -> (279.4128, -62.253)
  line L11 (279.4128, -62.253) -> (279.4128, -76.2523)
  line L12 (51.1005, -76.2523) -> (51.1005, -62.253)
  line L13 (51.1005, -62.253) -> (65.0998, -62.253)
  line L14 (65.0998, -62.253) -> (65.0998, -76.2523)
  line L15 (65.0998, -76.2523) -> (51.1005, -76.2523)
  line L16 (270.1758, -38.1522) -> (270.1758, -24.1528)
  line L17 (270.1758, -24.1528) -> (284.1748, -24.1528)
  line L18 (284.1748, -24.1528) -> (284.1748, -38.1522)
  line L19 (284.1748, -38.1522) -> (270.1758, -38.1522)
  line L20 (103.4878, -24.1528) -> (117.4878, -24.1528)
  line L21 (117.4878, -24.1528) -> (117.4878, -38.1522)
  line L22 (117.4878, -38.1522) -> (103.4878, -38.1522)
  line L23 (103.4878, -38.1522) -> (103.4878, -24.1528)
  line L24 (141.5878, -38.1522) -> (141.5878, -24.1528)
  line L25 (141.5878, -24.1528) -> (155.5878, -24.1528)
  line L26 (155.5878, -24.1528) -> (155.5878, -38.1522)
  line L27 (155.5878, -38.1522) -> (141.5878, -38.1522)
  line L28 (179.6878, -24.1528) -> (193.6878, -24.1528)
  line L29 (193.6878, -24.1528) -> (193.6878, -38.1522)
  line L30 (193.6878, -38.1522) -> (179.6878, -38.1522)
  line L31 (179.6878, -38.1522) -> (179.6878, -24.1528)
  line L32 (141.2998, -62.253) -> (141.2998, -76.2523)
  line L33 (141.2998, -76.2523) -> (127.3008, -76.2523)
  line L34 (127.3008, -76.2523) -> (127.3008, -62.253)
  line L35 (127.3008, -62.253) -> (141.2998, -62.253)
  line L36 (281.3678, -42.4519) -> (281.3678, -56.6526)
  line L37 (281.3678, -56.6526) -> (273.7928, -56.6526)
  line L38 (273.7928, -56.6526) -> (273.7928, -42.4519)
  line L39 (273.7928, -42.4519) -> (281.3678, -42.4519)
  line L40 (112.7248, -95.3023) -> (98.7241, -95.3023)
  line L41 (98.7241, -95.3023) -> (98.7241, -81.303)
  line L42 (98.7241, -81.303) -> (112.7248, -81.303)
  line L43 (112.7248, -81.303) -> (112.7248, -95.3023)
  line L44 (258.2678, -57.2023) -> (258.2678, -43.203)
  line L45 (258.2678, -43.203) -> (272.2688, -43.203)
  line L46 (272.2688, -43.203) -> (272.2688, -57.2023)
  line L47 (272.2688, -57.2023) -> (258.2678, -57.2023)
  line L48 (8.2379, -5.1029) -> (22.2375, -5.1029)
  line L49 (22.2375, -5.1029) -> (22.2375, -19.1023)
  line L50 (22.2375, -19.1023) -> (8.2379, -19.1023)
  line L51 (8.2379, -19.1023) -> (8.2379, -5.1029)
  line L52 (108.2508, -62.253) -> (122.2498, -62.253)
  line L53 (122.2498, -62.253) -> (122.2498, -76.2523)
  line L54 (122.2498, -76.2523) -> (108.2508, -76.2523)
  line L55 (108.2508, -76.2523) -> (108.2508, -62.253)
  line L56 (188.9248, -95.3023) -> (174.9258, -95.3023)
  line L57 (174.9258, -95.3023) -> (174.9258, -81.303)
  line L58 (174.9258, -81.303) -> (188.9248, -81.303)
  line L59 (188.9248, -81.303) -> (188.9248, -95.3023)
  line L60 (22.2375, -62.253) -> (22.2375, -76.2523)
  line L61 (22.2375, -76.2523) -> (8.2379, -76.2523)
  line L62 (8.2379, -76.2523) -> (8.2379, -62.253)
  line L63 (8.2379, -62.253) -> (22.2375, -62.253)
  line L64 (284.1748, -19.1023) -> (270.1758, -19.1023)
  line L65 (270.1758, -19.1023) -> (270.1758, -5.1029)
  line L66 (270.1758, -5.1029) -> (284.1748, -5.1029)
  line L67 (284.1748, -5.1029) -> (284.1748, -19.1023)
  line L68 (165.1128, -43.203) -> (165.1128, -57.2023)
  line L69 (165.1128, -57.2023) -> (151.1128, -57.2023)
  line L70 (151.1128, -57.2023) -> (151.1128, -43.203)
  line L71 (151.1128, -43.203) -> (165.1128, -43.203)
  line L72 (193.9758, -95.3023) -> (193.9758, -81.303)
  line L73 (193.9758, -81.303) -> (207.9748, -81.303)
  line L74 (207.9748, -81.303) -> (207.9748, -95.3023)
  line L75 (207.9748, -95.3023) -> (193.9758, -95.3023)
  line L76 (289.2258, -5.1029) -> (303.2248, -5.1029)
  line L77 (303.2248, -5.1029) -> (303.2248, -19.1023)
  line L78 (303.2248, -19.1023) -> (289.2258, -19.1023)
  line L79 (289.2258, -19.1023) -> (289.2258, -5.1029)
  line L80 (289.2258, -76.2523) -> (289.2258, -62.253)
  line L81 (289.2258, -62.253) -> (303.2248, -62.253)
  line L82 (303.2248, -62.253) -> (303.2248, -76.2523)
  line L83 (303.2248, -76.2523) -> (289.2258, -76.2523)
  line L84 (69.8623, -43.203) -> (69.8623, -57.2023)
  line L85 (69.8623, -57.2023) -> (55.863, -57.2023)
  line L86 (55.863, -57.2023) -> (55.863, -43.203)
  line L87 (55.863, -43.203) -> (69.8623, -43.203)
  line L88 (189.2128, -43.203) -> (203.2128, -43.203)
  line L89 (203.2128, -43.203) -> (203.2128, -57.2023)
  line L90 (203.2128, -57.2023) -> (189.2128, -57.2023)
  line L91 (189.2128, -57.2023) -> (189.2128, -43.203)
  line L92 (249.1688, -56.6526) -> (249.1688, -42.4519)
  line L93 (249.1688, -42.4519) -> (256.7438, -42.4519)
  line L94 (256.7438, -42.4519) -> (256.7438, -56.6526)
  line L95 (256.7438, -56.6526) -> (249.1688, -56.6526)
  line L96 (46.338, -24.1528) -> (60.3373, -24.1528)
  line L97 (60.3373, -24.1528) -> (60.3373, -38.1522)
  line L98 (60.3373, -38.1522) -> (46.338, -38.1522)
  line L99 (46.338, -38.1522) -> (46.338, -24.1528)
  line L100 (270.1758, -95.3023) -> (270.1758, -81.303)
  line L101 (270.1758, -81.303) -> (284.1748, -81.303)
  line L102 (284.1748, -81.303) -> (284.1748, -95.3023)
  line L103 (284.1748, -95.3023) -> (270.1758, -95.3023)
  line L104 (15.3817, -38.1522) -> (15.3817, -24.1528)
  line L105 (15.3817, -24.1528) -> (29.3812, -24.1528)
  line L106 (29.3812, -24.1528) -> (29.3812, -38.1522)
  line L107 (29.3812, -38.1522) -> (15.3817, -38.1522)
  line L108 (79.3873, -38.1522) -> (65.388, -38.1522)
  line L109 (65.388, -38.1522) -> (65.388, -24.1528)
  line L110 (65.388, -24.1528) -> (79.3873, -24.1528)
  line L111 (79.3873, -24.1528) -> (79.3873, -38.1522)
  line L112 (30.9067, -37.604) -> (30.9067, -23.4018)
  line L113 (30.9067, -23.4018) -> (38.4817, -23.4018)
  line L114 (38.4817, -23.4018) -> (38.4817, -37.604)
  line L115 (38.4817, -37.604) -> (30.9067, -37.604)
  line L116 (50.8123, -43.203) -> (50.8123, -57.2023)
  line L117 (50.8123, -57.2023) -> (36.813, -57.2023)
  line L118 (36.813, -57.2023) -> (36.813, -43.203)
  line L119 (36.813, -43.203) -> (50.8123, -43.203)
  line L120 (88.9123, -43.203) -> (88.9123, -57.2023)
  line L121 (88.9123, -57.2023) -> (74.913, -57.2023)
  line L122 (74.913, -57.2023) -> (74.913, -43.203)
  line L123 (74.913, -43.203) -> (88.9123, -43.203)
  line L124 (32.0505, -62.253) -> (46.0498, -62.253)
  line L125 (46.0498, -62.253) -> (46.0498, -76.2523)
  line L126 (46.0498, -76.2523) -> (32.0505, -76.2523)
  line L127 (32.0505, -76.2523) -> (32.0505, -62.253)
  line L128 (205.1748, -4.3518) -> (205.1748, -18.5539)
  line L129 (205.1748, -18.5539) -> (197.5998, -18.5539)
  line L130 (197.5998, -18.5539) -> (197.5998, -4.3518)
  line L131 (197.5998, -4.3518) -> (205.1748, -4.3518)
  line L132 (203.5008, -62.253) -> (217.4998, -62.253)
  line L133 (217.4998, -62.253) -> (217.4998, -76.2523)
  line L134 (217.4998, -76.2523) -> (203.5008, -76.2523)
  line L135 (203.5008, -76.2523) -> (203.5008, -62.253)
  line L136 (198.7378, -24.1528) -> (212.7378, -24.1528)
  line L137 (212.7378, -24.1528) -> (212.7378, -38.1522)
  line L138 (212.7378, -38.1522) -> (198.7378, -38.1522)
  line L139 (198.7378, -38.1522) -> (198.7378, -24.1528)
  line L140 (179.3998, -62.253) -> (179.3998, -76.2523)
  line L141 (179.3998, -76.2523) -> (165.4008, -76.2523)
  line L142 (165.4008, -76.2523) -> (165.4008, -62.253)
  line L143 (165.4008, -62.253) -> (179.3998, -62.253)
  line L144 (93.963, -57.2023) -> (93.963, -43.203)
  line L145 (93.963, -43.203) -> (107.9628, -43.203)
  line L146 (107.9628, -43.203) -> (107.9628, -57.2023)
  line L147 (107.9628, -57.2023) -> (93.963, -57.2023)
  line L148 (41.5755, -81.303) -> (55.5748, -81.303)
  line L149 (55.5748, -81.303) -> (55.5748, -95.3023)
  line L150 (55.5748, -95.3023) -> (41.5755, -95.3023)
  line L151 (41.5755, -95.3023) -> (41.5755, -81.303)
  line L152 (265.1248, -81.303) -> (265.1248, -95.3023)
  line L153 (265.1248, -95.3023) -> (251.1258, -95.3023)
  line L154 (251.1258, -95.3023) -> (251.1258, -81.303)
  line L155 (251.1258, -81.303) -> (265.1248, -81.303)
  line L156 (74.6248, -95.3023) -> (60.6255, -95.3023)
  line L157 (60.6255, -95.3023) -> (60.6255, -81.303)
  line L158 (60.6255, -81.303) -> (74.6248, -81.303)
  line L159 (74.6248, -81.303) -> (74.6248, -95.3023)
  line L160 (103.4382, -13.4529) -> (103.4382, -9.4529)
  line L161 (103.4382, -9.4529) -> (111.2021, -9.4529)
  arc A0 (115.6743, -9.4529) -> (111.2021, -9.4529) centre (113.4382, -11.4529) ccw
  line L162 (115.6743, -9.4529) -> (123.4382, -9.4529)
  line L163 (123.4382, -9.4529) -> (123.4382, -13.4529)
  line L164 (123.4382, -13.4529) -> (115.6743, -13.4529)
  arc A1 (111.2021, -13.4529) -> (115.6743, -13.4529) centre (113.4382, -11.4529) ccw
  line L165 (111.2021, -13.4529) -> (103.4382, -13.4529)
  line L166 (217.7878, -5.1029) -> (231.7878, -5.1029)
  line L167 (231.7878, -5.1029) -> (231.7878, -19.1023)
  line L168 (231.7878, -19.1023) -> (217.7878, -19.1023)
  line L169 (217.7878, -19.1023) -> (217.7878, -5.1029)
  line L170 (241.6008, -62.253) -> (255.5998, -62.253)
  line L171 (255.5998, -62.253) -> (255.5998, -76.2523)
  line L172 (255.5998, -76.2523) -> (241.6008, -76.2523)
  line L173 (241.6008, -76.2523) -> (241.6008, -62.253)
  line L174 (136.8258, -95.3023) -> (136.8258, -81.303)
  line L175 (136.8258, -81.303) -> (150.8248, -81.303)
  line L176 (150.8248, -81.303) -> (150.8248, -95.3023)
  line L177 (150.8248, -95.3023) -> (136.8258, -95.3023)
  line L178 (122.5378, -38.1522) -> (122.5378, -24.1528)
  line L179 (122.5378, -24.1528) -> (136.5378, -24.1528)
  line L180 (136.5378, -24.1528) -> (136.5378, -38.1522)
  line L181 (136.5378, -38.1522) -> (122.5378, -38.1522)
  line L182 (184.1628, -43.203) -> (184.1628, -57.2023)
  line L183 (184.1628, -57.2023) -> (170.1628, -57.2023)
  line L184 (170.1628, -57.2023) -> (170.1628, -43.203)
  line L185 (170.1628, -43.203) -> (184.1628, -43.203)
  line L186 (208.2628, -43.203) -> (222.2628, -43.203)
  line L187 (222.2628, -43.203) -> (222.2628, -57.2023)
  line L188 (222.2628, -57.2023) -> (208.2628, -57.2023)
  line L189 (208.2628, -57.2023) -> (208.2628, -43.203)
  line L190 (84.1498, -76.2523) -> (70.1505, -76.2523)
  line L191 (70.1505, -76.2523) -> (70.1505, -62.253)
  line L192 (70.1505, -62.253) -> (84.1498, -62.253)
  line L193 (84.1498, -62.253) -> (84.1498, -76.2523)
  line L194 (257.9808, -24.1528) -> (257.9808, -38.1522)
  line L195 (257.9808, -38.1522) -> (243.9818, -38.1522)
  line L196 (243.9818, -38.1522) -> (243.9818, -24.1528)
  line L197 (243.9818, -24.1528) -> (257.9808, -24.1528)
  line L198 (113.0128, -43.203) -> (127.0128, -43.203)
  line L199 (127.0128, -43.203) -> (127.0128, -57.2023)
  line L200 (127.0128, -57.2023) -> (113.0128, -57.2023)
  line L201 (113.0128, -57.2023) -> (113.0128, -43.203)
  line L202 (184.4508, -62.253) -> (198.4498, -62.253)
  line L203 (198.4498, -62.253) -> (198.4498, -76.2523)
  line L204 (198.4498, -76.2523) -> (184.4508, -76.2523)
  line L205 (184.4508, -76.2523) -> (184.4508, -62.253)
  line L206 (69.8623, -5.1029) -> (69.8623, -19.1023)
  line L207 (69.8623, -19.1023) -> (55.863, -19.1023)
  line L208 (55.863, -19.1023) -> (55.863, -5.1029)
  line L209 (55.863, -5.1029) -> (69.8623, -5.1029)
  line L210 (265.1248, -5.1029) -> (265.1248, -19.1023)
  line L211 (265.1248, -19.1023) -> (251.1258, -19.1023)
  line L212 (251.1258, -19.1023) -> (251.1258, -5.1029)
  line L213 (251.1258, -5.1029) -> (265.1248, -5.1029)
  line L214 (82.4755, -4.3518) -> (90.0507, -4.3518)
  line L215 (90.0507, -4.3518) -> (90.0507, -18.5539)
  line L216 (90.0507, -18.5539) -> (82.4755, -18.5539)
  line L217 (82.4755, -18.5539) -> (82.4755, -4.3518)
  line L218 (36.5248, -95.3023) -> (22.5255, -95.3023)
  line L219 (22.5255, -95.3023) -> (22.5255, -81.303)
  line L220 (22.5255, -81.303) -> (36.5248, -81.303)
  line L221 (36.5248, -81.303) -> (36.5248, -95.3023)
  line L222 (160.3498, -62.253) -> (160.3498, -76.2523)
  line L223 (160.3498, -76.2523) -> (146.3508, -76.2523)
  line L224 (146.3508, -76.2523) -> (146.3508, -62.253)
  line L225 (146.3508, -62.253) -> (160.3498, -62.253)
  line L226 (160.6378, -24.1528) -> (174.6378, -24.1528)
  line L227 (174.6378, -24.1528) -> (174.6378, -38.1522)
  line L228 (174.6378, -38.1522) -> (160.6378, -38.1522)
  line L229 (160.6378, -38.1522) -> (160.6378, -24.1528)
  line L230 (184.2123, -9.4529) -> (184.2123, -13.4529)
  line L231 (184.2123, -13.4529) -> (176.4484, -13.4529)
  arc A2 (171.9762, -13.4529) -> (176.4484, -13.4529) centre (174.2123, -11.4529) ccw
  line L232 (171.9762, -13.4529) -> (164.2123, -13.4529)
  line L233 (164.2123, -13.4529) -> (164.2123, -9.4529)
  line L234 (164.2123, -9.4529) -> (171.9762, -9.4529)
  arc A3 (176.4484, -9.4529) -> (171.9762, -9.4529) centre (174.2123, -11.4529) ccw
  line L235 (176.4484, -9.4529) -> (184.2123, -9.4529)
  line L236 (131.7748, -95.3023) -> (117.7738, -95.3023)
  line L237 (117.7738, -95.3023) -> (117.7738, -81.303)
  line L238 (117.7738, -81.303) -> (131.7748, -81.303)
  line L239 (131.7748, -81.303) -> (131.7748, -95.3023)
  line L240 (103.1998, -76.2523) -> (89.2005, -76.2523)
  line L241 (89.2005, -76.2523) -> (89.2005, -62.253)
  line L242 (89.2005, -62.253) -> (103.1998, -62.253)
  line L243 (103.1998, -62.253) -> (103.1998, -76.2523)
  line L244 (6.2811, -37.604) -> (6.2811, -23.4018)
  line L245 (6.2811, -23.4018) -> (13.8562, -23.4018)
  line L246 (13.8562, -23.4018) -> (13.8562, -37.604)
  line L247 (13.8562, -37.604) -> (6.2811, -37.604)
  line L248 (241.3128, -57.2023) -> (227.3128, -57.2023)
  line L249 (227.3128, -57.2023) -> (227.3128, -43.203)
  line L250 (227.3128, -43.203) -> (241.3128, -43.203)
  line L251 (241.3128, -43.203) -> (241.3128, -57.2023)
  line L252 (150.8248, -19.1023) -> (136.8258, -19.1023)
  line L253 (136.8258, -19.1023) -> (136.8258, -5.1029)
  line L254 (136.8258, -5.1029) -> (150.8248, -5.1029)
  line L255 (150.8248, -5.1029) -> (150.8248, -19.1023)
  line L256 (289.2258, -43.203) -> (303.2248, -43.203)
  line L257 (303.2248, -43.203) -> (303.2248, -57.2023)
  line L258 (303.2248, -57.2023) -> (289.2258, -57.2023)
  line L259 (289.2258, -57.2023) -> (289.2258, -43.203)
  line L260 (217.7878, -38.1522) -> (217.7878, -24.1528)
  line L261 (217.7878, -24.1528) -> (231.7878, -24.1528)
  line L262 (231.7878, -24.1528) -> (231.7878, -38.1522)
  line L263 (231.7878, -38.1522) -> (217.7878, -38.1522)
  line L264 (227.0248, -81.303) -> (227.0248, -95.3023)
  line L265 (227.0248, -95.3023) -> (213.0258, -95.3023)
  line L266 (213.0258, -95.3023) -> (213.0258, -81.303)
  line L267 (213.0258, -81.303) -> (227.0248, -81.303)
  line L268 (24.6187, -57.2023) -> (10.6178, -57.2023)
  line L269 (10.6178, -57.2023) -> (10.6178, -43.203)
  line L270 (10.6178, -43.203) -> (24.6187, -43.203)
  line L271 (24.6187, -43.203) -> (24.6187, -57.2023)
  line L272 (232.0758, -95.3023) -> (232.0758, -81.303)
  line L273 (232.0758, -81.303) -> (246.0748, -81.303)
  line L274 (246.0748, -81.303) -> (246.0748, -95.3023)
  line L275 (246.0748, -95.3023) -> (232.0758, -95.3023)
  line L276 (146.0628, -43.203) -> (146.0628, -57.2023)
  line L277 (146.0628, -57.2023) -> (132.0628, -57.2023)
  line L278 (132.0628, -57.2023) -> (132.0628, -43.203)
  line L279 (132.0628, -43.203) -> (146.0628, -43.203)
  line L280 (236.5498, -76.2523) -> (222.5508, -76.2523)
  line L281 (222.5508, -76.2523) -> (222.5508, -62.253)
  line L282 (222.5508, -62.253) -> (236.5498, -62.253)
  line L283 (236.5498, -62.253) -> (236.5498, -76.2523)
  line L284 (155.8758, -81.303) -> (169.8748, -81.303)
  line L285 (169.8748, -81.303) -> (169.8748, -95.3023)
  line L286 (169.8748, -95.3023) -> (155.8758, -95.3023)
  line L287 (155.8758, -95.3023) -> (155.8758, -81.303)
  line L288 (93.6748, -81.303) -> (93.6748, -95.3023)
  line L289 (93.6748, -95.3023) -> (79.6755, -95.3023)
  line L290 (79.6755, -95.3023) -> (79.6755, -81.303)
  line L291 (79.6755, -81.303) -> (93.6748, -81.303)
  line L292 (289.2258, -38.1522) -> (289.2258, -24.1528)
  line L293 (289.2258, -24.1528) -> (303.2248, -24.1528)
  line L294 (303.2248, -24.1528) -> (303.2248, -38.1522)
  line L295 (303.2248, -38.1522) -> (289.2258, -38.1522)
  line L296 (-5.4742, -104.2517) -> (312.1758, -104.2517)
  line L297 (312.1758, -104.2517) -> (312.1758, 3.8481)
  line L298 (312.1758, 3.8481) -> (-5.4742, 3.8481)
  line L299 (-5.4742, 3.8481) -> (-5.4742, -104.2517)
  line L300 (277.1753, -95.3023) -> (274.6753, -95.3023)
  line L301 (274.6753, -95.3023) -> (274.6753, -95.8023)
  line L302 (274.6753, -95.8023) -> (277.1753, -95.8023)